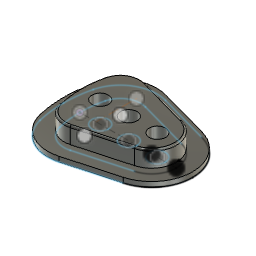
xl10_camera_mount_22mm (Autodesk Fusion 360 design; units mm, degrees)
Autodesk Fusion 360 part; units mm, degrees
sketch "Sketch1" plane through (0, 0, 0) normal (0, 0, 1) x (1, 0, 0)
  line L0 (0, 0) -> (11.8, 0) construction
  line L1 (2, 0) -> (2, 4.9481) construction
  line L2 (9.6021, 2.8908) -> (3.4309, 4.603)
  arc A0 (0.3331, 2.7838) -> (0, 0) centre (11.8, 0) ccw
  arc A1 (11.8, 0) -> (9.6021, 2.8908) centre (8.8, 0) ccw
  arc A2 (3.4309, 4.603) -> (0.3331, 2.7838) centre (2.7625, 2.194) ccw
  arc A3 (0, 0) -> (0.3331, -2.7838) centre (11.8, 0) ccw
  arc A4 (0.3331, -2.7838) -> (3.4309, -4.603) centre (2.7625, -2.194) ccw
  line L3 (9.6021, -2.8908) -> (3.4309, -4.603)
  arc A5 (9.6021, -2.8908) -> (11.8, 0) centre (8.8, 0) ccw
  circle A6 centre (6, 0) radius 1
  circle A7 centre (2.5, 0) radius 1
  circle A8 centre (9.5, 0) radius 1
  arc A9 (-2, 0) -> (-1.6105, -3.2556) centre (11.8, 0) ccw
  arc A10 (-1.6105, -3.2556) -> (3.9656, -6.5302) centre (2.7625, -2.194) ccw
  line L4 (10.1368, -4.818) -> (3.9656, -6.5302)
  arc A11 (10.1368, -4.818) -> (13.8, 0) centre (8.8, 0) ccw
  arc A12 (13.8, 0) -> (10.1368, 4.818) centre (8.8, 0) ccw
  line L5 (10.1368, 4.818) -> (3.9656, 6.5302)
  arc A13 (3.9656, 6.5302) -> (-1.6105, 3.2556) centre (2.7625, 2.194) ccw
  arc A14 (-1.6105, 3.2556) -> (-2, 0) centre (11.8, 0) ccw
  dimension "d1" = 11.8
  dimension "d2" = 6
  dimension "d4" = 5
  dimension "d5" = 2
  dimension "d6" = 6
  dimension "d7" = 2
  dimension "d8" = 2.5
  dimension "d9" = 2
  dimension "d10" = 3.5
  dimension "d11" = 2
  constraint coincident L0.start A0.end
  constraint horizontal L0
  constraint coincident L0 A1.centre
  constraint coincident L0 L1.start
  constraint perpendicular L0 L1
  constraint coincident L0.end A0.centre
  constraint coincident L0 A0.end
  constraint tangent A0 A2
  constraint symmetric A0.centre L0 A1.start
  constraint symmetric L0 L2.start L3.start
  constraint symmetric L0 A0 A3
  constraint symmetric L0 A0.end A3.start
  constraint symmetric L0 A1 A5
  constraint symmetric L0 L2.end A4.end
  constraint symmetric L0 A0.start A3.end
  constraint symmetric L0 A2 A4
  constraint coincident L0 A6.centre
  constraint coincident L0 A7.centre
  constraint coincident L0 A8.centre
  measures "d1" distance of L0.start L0.end
  measures "d2" diameter of A1
  measures "d4" diameter of A2
  measures "d5" diameter of A6
  measures "d6" distance of L0.start A6.centre
  measures "d7" diameter of A7
  measures "d8" distance of L0.start A7.centre
  measures "d9" diameter of A8
  measures "d10" distance of A6.centre A8.centre
extrude "Extrude1" add sketch "Sketch1" along normal blind 2.6 contours L2 A0 A1 A2 A3 A4 L3 A5
extrude "Extrude2" add sketch "Sketch1" along normal blind 0.6 contours A9 A10 L4 A11 A12 L5 A13 A14
fillet "Fillet1" radius 0.2 6 edges at (6.5165, 3.7469, 2.6) (1.4965, 4.3498, 2.6) (0, 0, 2.6) (1.4965, -4.3498, 2.6) (6.5165, -3.7469, 2.6) (11.8, 0, 2.6)
